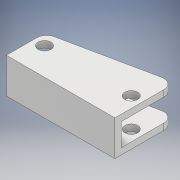
# Autodesk Inventor part: finger1
Saved by Autodesk Inventor 2018 (Build 220112000, 112)
## iProperties
Created: 2018-02-19
Part Number: finger1
Material: Plastique ABS
Document SubType Name: Modeling
Designer: Thomas
Density: 1.06 g/cm^3
Appearance: Lisse - Blanc
Author: Thomas
Autodesk Inventor part; units mm, degrees
ref_plane "YZ Plane" through (0, 0, 0) normal (1, 0, 0) x (0, 1, 0)
ref_plane "XZ Plane" through (0, 0, 0) normal (0, 1, 0) x (-1, 0, 0)
ref_plane "XY Plane" through (0, 0, 0) normal (0, 0, 1) x (1, 0, 0)
sketch "Esquisse1" plane through (0, 0, 0) normal (0, 0, 1) x (1, 0, 0)
  line L0 (0, 0) -> (33.8, 0)
  line L1 (0, 0) -> (0, 9.5191)
  line L2 (2.3899, 12.4564) -> (30.1899, 18.2302)
  line L3 (33.8, 15.2929) -> (33.8, 0)
  arc A0 (2.3899, 12.4564) -> (0, 9.5191) centre (3, 9.5191) ccw
  arc A1 (33.8, 15.2929) -> (30.1899, 18.2302) centre (30.8, 15.2929) ccw
  point P0 (0, 11.96)
  point P1 (33.8, 18.98)
  dimension "d0" = 33.8
  dimension "d1" = 18.98
  dimension "d2" = 11.96
  dimension "d3" = 3
  dimension "d4" = 3
  constraints: 8 end point, 4 point on circle, 4 point on line, 4 tangent, 2 centre point, 1 horizontal, 1 parallel, 1 vertical
  measures "d0" distance of L0.start L0.end
  measures "d1" distance of point (33.8, 18.98) L0.end
  measures "d2" distance of L0.start point (0, 11.96)
  measures "d3" radius of A0
  measures "d4" radius of A1
extrude "Extrusion1" add sketch "Esquisse1" against normal blind 2
sketch "Esquisse2" plane through (0, 0, 0) normal (0, -1, 0) x (1, 0, 0)
  line L0 (33.8, -2) -> (0, -2) projected
  line L1 (33.8, -2) -> (0, -2)
  line L2 (0, -2) -> (0, -11)
  line L3 (0, -11) -> (33.8, -11)
  line L4 (33.8, -11) -> (33.8, -2)
  point P0 (33.8, 0)
  dimension "d8" = 9
  constraints: 8 end point, 2 parallel, 1 horizontal, 1 perpendicular
  measures "d8" distance of L1.end L2.end
extrude "Extrusion2" add sketch "Esquisse2" against normal blind 2
sketch "Esquisse3" plane through (33.8, 0, -11) normal (0, 0, -1) x (-1, 0, 0)
  line L0 (0, 2) -> (33.8, 2) projected
  line L1 (33.8, 2) -> (33.8, 9.5191)
  line L2 (0, 15.2929) -> (0, 2) projected
  line L3 (0, 15.2929) -> (0, 2)
  line L4 (0, 2) -> (33.8, 2)
  line L5 (3.6101, 18.2302) -> (31.4101, 12.4564)
  arc A0 (3.6101, 18.2302) -> (0, 15.2929) centre (3, 15.2929) ccw
  arc A1 (33.8, 9.5191) -> (31.4101, 12.4564) centre (30.8, 9.5191) ccw
  point P0 (33.8, 0)
  point P1 (33.8, 11.96)
  point P2 (0, 18.98)
  dimension "d11" = 9.96
  dimension "d12" = 16.98
  dimension "d13" = 3
  constraints: 8 end point, 4 point on circle, 4 point on line, 4 tangent, 2 centre point, 1 equal radius, 1 parallel, 1 perpendicular, 1 vertical
  measures "d11" distance of L0.end point (33.8, 11.96)
  measures "d12" distance of point (0, 18.98) L0.start
  measures "d13" radius of A0
extrude "Extrusion3" add sketch "Esquisse3" against normal blind 2
sketch "Esquisse4" plane through (0, 0, 0) normal (0, 0, 1) x (1, 0, 0)
  line L0 (0, 0) -> (3.39, 0) construction
  line L1 (0, 0) -> (33.8, 0) construction
  line L2 (3.39, 8.5) -> (3.39, 0) construction
  circle A0 centre (3.39, 8.5) radius 2
  circle A1 centre (30.41, 8.5) radius 2
  line L3 (33.8, 0) -> (33.8, 15.2929) projected
  dimension "d16" = 3.39
  dimension "d17" = 8.5
  dimension "d19" = 4
  dimension "d20" = 4
  dimension "d21" = 3.39
  dimension "d26" = 8.5
  constraints: 4 end point, 2 centre point, 1 coincident, 1 perpendicular, 1 point on line
  measures "d16" distance of L0.start L0.end
  measures "d17" distance of L2.start L0.end
  measures "d19" diameter of A0
  measures "d20" diameter of A1
  measures "d21" distance from line of L3 A1.centre
  measures "d26" distance from line of L1 A1.centre
extrude "Extrusion4" cut sketch "Esquisse4" against normal blind 2
sketch "Esquisse5" plane through (33.8, 0, -11) normal (0, 0, -1) x (-1, 0, 0)
  circle A0 centre (3.39, 8.5) radius 2 projected
  circle A1 centre (3.39, 8.5) radius 2
  circle A2 centre (30.41, 8.5) radius 2 projected
  circle A3 centre (30.41, 8.5) radius 2
  point P0 (33.8, 0)
  constraints: 2 centre point, 2 coincident, 1 concentric
extrude "Extrusion5" cut sketch "Esquisse5" against normal blind 2
